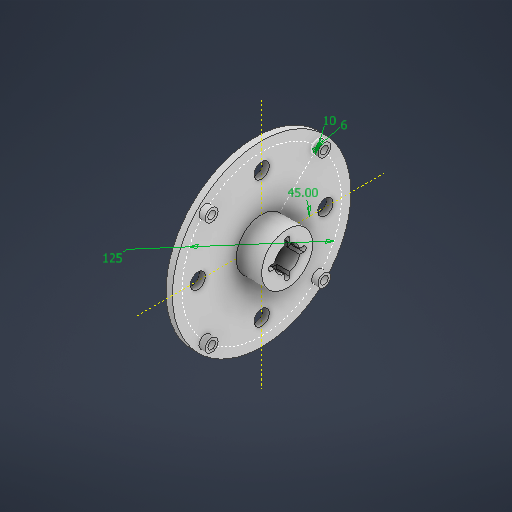
# Autodesk Inventor part: Hub
Saved by Autodesk Inventor 2026.1 (Build 301233000, 233)
## iProperties
Created: 2026-06-12
Part Number: Hub
Material: Generic
Document SubType Name: Modeling
Designer: share
Density: 1 g/cm^3
Appearance: Default
Author: share
Autodesk Inventor part; units mm, degrees
ref_plane "YZ Plane" through (0, 0, 0) normal (1, 0, 0) x (0, 1, 0)
ref_plane "XY Plane" through (0, 0, 0) normal (0, 0, 1) x (1, 0, 0)
sketch "Sketch1" plane through (0, 0, 0) normal (1, 0, 0) x (0, 1, 0)
  circle A0 centre (0, 0) radius 70
  dimension "d2" = 140
  constraints: 1 centre point, 1 coincident
  measures "d2" diameter of A0
extrude "Hub Face" add sketch "Sketch1" along normal blind 5
sketch "Sketch2" plane through (5, 0, 0) normal (1, 0, 0) x (0, 0, -1)
  circle A0 centre (0, 0) radius 50 construction
  circle A1 centre (0, 50) radius 6
  line L0 (0, 50) -> (0, 0) construction
  dimension "d4" = 100
  dimension "d3" = 12
  constraints: 2 end point, 1 centre point, 1 coincident, 1 vertical, 1 vertical alignment, 2 other
  measures "d3" diameter of A1
extrude "Lug Bolt Hole" cut sketch "Sketch2" against normal up to surface (5 mm away)
pattern_circular "Lug Bolt Hole Pattern" count 4 over 360 about axis through (-10, 0, 0) along (1, 0, 0) of "Lug Bolt Hole"
sketch "Sketch3" plane through (5, 0, 0) normal (1, 0, 0) x (0, 0, -1)
  circle A0 centre (0, 0) radius 20
  circle A1 centre (0, 0) radius 10
  line L0 (-98, 0) -> (98, 0) construction
  line L1 (0, -98) -> (0, 98) construction
  arc A2 (13, -2) -> (13, 2) centre (13, 0) ccw
  arc A3 (7, 2) -> (7, -2) centre (7, 0) ccw
  line L2 (13, 2) -> (7, 2)
  line L3 (13, -2) -> (7, -2)
  point P0 (10, 0)
  point P1 (9.798, -2)
  point P2 (9.798, 2)
  dimension "d19" = 20
  dimension "d10" = 40
  dimension "d59" = 6
  dimension "d60" = 2
  dimension "d61" = 7
  dimension "d62" = 3
  dimension "d63" = 3
  constraints: 4 end point, 4 point on circle, 3 centre point, 3 point on line, 2 coincident, 2 tangent, 1 equal radius, 1 horizontal, 1 parallel, 3 other
  measures "d10" diameter of A0
  measures "d59" distance of A3.centre A2.centre
  measures "d60" radius of A2
  measures "d61" distance from line of L1 A3.centre
  measures "d62" distance of A3.centre point (10, 0)
  measures "d63" distance of point (10, 0) A2.centre
extrude "Hub Shaft" add sketch "Sketch3" along normal blind 20 contours A0 | A1 L2 A2 L3
ref_plane "Lock Pin Hole Plane" through (0, 15.875, 0) normal (0, 1, 0) x (-1, 0, 0)
sketch "Sketch10" plane through (25, 0, 0) normal (1, 0, 0) x (0, 0, -1)
  line L0 (-98, 0) -> (98, 0) construction
  arc A0 (7, 2) -> (7, -2) centre (7, 0) ccw projected
  line L1 (13, 2) -> (7, 2) projected
  line L2 (13, -2) -> (7, -2) projected
  arc A1 (13, -2) -> (13, 2) centre (13, 0) ccw projected
  point P0 (0, 0)
  dimension "d75" = 6
  dimension "d76" = 2
  measures "d75" distance of A1.centre A0.centre
  measures "d76" radius of A1
extrude "Key Slot" cut sketch "Sketch10" against normal blind 10
pattern_circular "Key Slot Pattern" count 4 over 360 about axis through (-10, 0, 0) along (1, 0, 0) of "Key Slot"
sketch "Sketch12" plane through (5, 0, 0) normal (1, 0, 0) x (0, 0, -1)
  arc A0 (-2, 9.798) -> (-9.798, 2) centre (0, 0) ccw construction
  arc A1 (-9.798, -2) -> (-2, -9.798) centre (0, 0) ccw construction
  arc A2 (2, -9.798) -> (9.798, -2) centre (0, 0) ccw construction
  arc A3 (9.798, 2) -> (2, 9.798) centre (0, 0) ccw construction
  circle A4 centre (0, 0) radius 10 construction
  circle A5 centre (0, 0) radius 10
  circle A6 centre (0, 0) radius 5
  dimension "d74" = 10
  constraints: 3 centre point, 3 coincident, 2 concentric
  measures "d74" diameter of A6
extrude "Extrusion10" cut sketch "Sketch12" against normal through all contours A6
sketch "Sketch13" plane through (0, 0, 0) normal (-1, 0, 0) x (0, 0, 1)
  circle A0 centre (0, 0) radius 15
  circle A1 centre (0, 0) radius 12.5
  dimension "d77" = 30
  dimension "d78" = 25
  constraints: 2 centre point, 2 coincident
  measures "d77" diameter of A0
  measures "d78" diameter of A1
extrude "Extrusion11" add sketch "Sketch13" along normal blind 3
sketch "Sketch14" plane through (5, 0, 0) normal (1, 0, 0) x (0, 0, -1)
  circle A0 centre (0, 0) radius 62.5 construction
  circle A1 centre (44.1942, 44.1942) radius 5
  line L0 (-98, 0) -> (98, 0) construction
  line L1 (0, -98) -> (0, 98) construction
  line L2 (0, 0) -> (44.1942, 44.1942) construction
  circle A2 centre (44.1942, 44.1942) radius 3
  dimension "d81" = 125
  dimension "d82" = 45
  dimension "d83" = 10
  dimension "d84" = 6
  constraints: 2 centre point, 2 coincident, 2 end point, 3 other
  measures "d82" angle of L0 L2
  measures "d83" diameter of A1
  measures "d84" diameter of A2
extrude "Extrusion12" add sketch "Sketch14" along normal blind 5
extrude "Extrusion13" cut sketch "Sketch14" against normal through all contours A2
pattern_circular "Circular Pattern6" count 4 over 360 about axis through (-10, 0, 0) along (1, 0, 0) of "Extrusion12", "Extrusion13"
equation "\"d2\" = Hub_Diameter"
equation "\"d0\" = Hub_Thickness"
equation "\"d4\" = Lug_Bolt_Pattern_Diameter"
equation "\"d3\" = Lug_Bolt_Hole_Diameter"
equation "\"d17\" = Hub_Shaft_Length"
equation "\"Hub_Thickness\" = 5"
equation "\"Hub_Diameter\" = 140"
equation "\"Lug_Bolt_Hole_Diameter\" = 12"
equation "\"Hub_Shaft_Diameter\" = 1"
equation "\"Hub_Shaft_Wall_Thickness\" = 1"
equation "\"Hub_Shaft_Length\" = 20"
equation "\"Hub_Shaft_Outer_Diameter\" = 31.75"
equation "\"d20\" = 0.5 * Hub_Shaft_Outer_Diameter"
equation "\"Lock_Pin_Edge_Distance\" = 15"
equation "\"Wheel_Center_Hub_Diameter_Wall_Thickness\" = 5"
equation "\"Wheel_Center_Hub_Length\" = 5"
equation "\"Weight_Reduction_Hole_Angle\" = 45deg"
equation "\"Lug_Bolt_Pattern_Diameter\" = 100"
body "Solid1"
